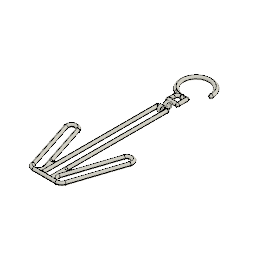
shoe-hanger v3 (Autodesk Fusion 360 design; units mm, degrees)
Autodesk Fusion 360 part; units mm, degrees
sketch "Sketch1" plane through (0, 0, 0) normal (0, 0, 1) x (1, 0, 0) in component "shoe holder"
  line L0 (67.4979, 112.1793) -> (43.75, 119.9918)
  line L1 (43.75, 119.9918) -> (12.5, 25)
  line L2 (12.5, 225) -> (-12.5, 225)
  line L3 (-12.5, 225) -> (-12.5, 25)
  line L4 (12.5, 25) -> (12.5, 225)
  line L5 (30.5937, 0) -> (-30.5937, 0)
  line L6 (0, 225) -> (0, 0) construction
  line L7 (67.4979, 112.1793) -> (30.5937, 0)
  line L8 (-67.4979, 112.1793) -> (-43.75, 119.9918)
  line L9 (-43.75, 119.9918) -> (-12.5, 25)
  line L10 (-67.4979, 112.1793) -> (-30.5937, 0)
  dimension "d8" = 25
  dimension "d11" = 25
  dimension "d14" = 200
  dimension "d56" = 100
  dimension "d57" = 100
  dimension "d58" = 31.25
  dimension "d59" = 25
  constraint horizontal L2
  constraint perpendicular L2 L3
  constraint parallel L3 L4
  constraint horizontal L5
  constraint midpoint L2 L6.start
  constraint coincident L6.end origin
  constraint symmetric L0.start L6 L8.start
  constraint symmetric L0.end L6 L8.end
  constraint parallel L9 L10
  constraint parallel L1 L7
  constraint perpendicular L0 L1
  constraint perpendicular L8 L9
  constraint coincident L1.end L4.start
  constraint midpoint L5 L6.end
  constraint coincident L3.end L9.end
  measures "d8" distance of L3.end L1.end
  measures "d11" distance of L0.start L0.end
  measures "d14" distance of L2.start L1.end
  measures "d56" distance of L0.end L1.end
  measures "d57" distance of L3.end L8.end
  measures "d58" distance of L0.end L4
  measures "d59" distance of L1.end L5
extrude "Extrude1" add sketch "Sketch1" along normal blind 8 makes body 1 in component "shoe holder"
fillet "Fillet1" radius 12.5 6 edges at (-67.4979, 112.1793, 4) (-43.75, 119.9918, 4) (-30.5937, 0, 4) (30.5937, 0, 4) (67.4979, 112.1793, 4) (43.75, 119.9918, 4) on bodies 1 in component "shoe holder"
fillet "Fillet1" radius 1.3333 2 edges at (-12.5, 25, 4) (12.5, 25, 4) on bodies 1 in component "shoe holder"
sketch "Sketch3" plane through (0, 0, 8) normal (0, 0, 1) x (-1, 0, 0) in component "shoe holder"
  arc A0 (-21.5468, 0) -> (-33.4208, -8.5938) centre (-21.5468, -12.5) ccw
  line L0 (-33.4208, -8.5938) -> (-63.5917, -100.3053)
  line L1 (-39.8438, -108.1178) -> (-15.0999, -32.903)
  line L2 (-12.5, -33.3196) -> (-12.5, -225)
  line L3 (12.5, -225) -> (12.5, -33.3196)
  line L4 (15.0999, -32.903) -> (39.8437, -108.1178)
  arc A1 (39.8437, -108.1178) -> (63.5917, -100.3053) centre (51.7177, -104.2116) ccw
  line L5 (63.5917, -100.3053) -> (33.4208, -8.5938)
  arc A2 (33.4208, -8.5938) -> (21.5468, 0) centre (21.5468, -12.5) ccw
  line L6 (21.5468, 0) -> (-21.5468, 0)
  arc A3 (26.2964, -10.9375) -> (16.7972, -14.0625) centre (21.5468, -12.5) ccw
  arc A4 (-21.5468, -7.5) -> (-26.2964, -10.9375) centre (-21.5468, -12.5) ccw
  line L7 (-26.2964, -10.9375) -> (-56.4673, -102.6491)
  arc A5 (-56.4673, -102.6491) -> (-46.9681, -105.7741) centre (-51.7177, -104.2116) ccw
  arc A6 (46.9681, -105.7741) -> (56.4673, -102.6491) centre (51.7177, -104.2116) ccw
  line L8 (56.4673, -102.6491) -> (26.2964, -10.9375)
  line L9 (46.9681, -105.7741) -> (16.7972, -14.0625)
  line L10 (-46.9681, -105.7741) -> (-16.7972, -14.0625)
  arc A7 (-16.7972, -14.0625) -> (-26.2964, -10.9375) centre (-21.5468, -12.5) ccw
  arc A8 (26.2964, -10.9375) -> (16.7972, -14.0625) centre (21.5468, -12.5) ccw
  arc A9 (-63.5917, -100.3053) -> (-39.8438, -108.1178) centre (-51.7177, -104.2116) ccw
  arc A10 (-12.5, -33.3196) -> (-15.0999, -32.903) centre (-13.8333, -33.3196) ccw
  arc A11 (15.0999, -32.903) -> (12.5, -33.3196) centre (13.8333, -33.3196) ccw
  dimension "d37" = 10
  dimension "d38" = 10
  constraint tangent A6 L9
  constraint tangent A5 L10
  constraint concentric A2 A3
  constraint concentric A0 A4
  constraint parallel L0 L7
  constraint concentric A1 A6
  constraint parallel L5 L8
  constraint tangent A3 L8
  constraint tangent A4 L7
  constraint tangent L7 A5
  constraint tangent A6 L8
  constraint concentric A3 A8
  constraint tangent L9 A8
  constraint concentric A4 A7
  measures "d37" distance of L8 L9
  measures "d38" distance of L7 L10
extrude "Extrude3" cut sketch "Sketch3" against normal through all bodies 1 in component "shoe holder"
sketch "Sketch4" plane through (0, 0, 8) normal (0, 0, 1) x (-1, 0, 0) in component "shoe holder"
  line L0 (46.9681, -105.7741) -> (16.7972, -14.0625)
  arc A0 (26.2964, -10.9375) -> (16.7972, -14.0625) centre (21.5468, -12.5) ccw
  line L1 (26.2964, -10.9375) -> (56.4673, -102.6491)
  arc A1 (46.9681, -105.7741) -> (56.4673, -102.6491) centre (51.7177, -104.2116) ccw
  line L2 (-16.7972, -14.0625) -> (-46.9681, -105.7741)
  arc A2 (-56.4673, -102.6491) -> (-46.9681, -105.7741) centre (-51.7177, -104.2116) ccw
  line L3 (-56.4673, -102.6491) -> (-26.2964, -10.9375)
  arc A3 (-16.7972, -14.0625) -> (-26.2964, -10.9375) centre (-21.5468, -12.5) ccw
  arc A4 (-21.5468, 0) -> (-33.4208, -8.5938) centre (-21.5468, -12.5) ccw
  line L4 (-33.4208, -8.5938) -> (-63.5917, -100.3053)
  line L5 (-39.8438, -108.1178) -> (-15.0999, -32.903)
  line L6 (-12.5, -33.3196) -> (-12.5, -225)
  line L7 (-12.5, -225) -> (12.5, -225)
  line L8 (12.5, -225) -> (12.5, -33.3196)
  line L9 (15.0999, -32.903) -> (39.8437, -108.1178)
  arc A5 (39.8437, -108.1178) -> (63.5917, -100.3053) centre (51.7177, -104.2116) ccw
  line L10 (63.5917, -100.3053) -> (33.4208, -8.5938)
  arc A6 (33.4208, -8.5938) -> (21.5468, 0) centre (21.5468, -12.5) ccw
  line L11 (21.5468, 0) -> (-21.5468, 0)
  line L12 (-4.5, -217) -> (4.5, -217)
  line L13 (-4.5, -217) -> (-4.5, -8)
  line L14 (4.5, -8) -> (-4.5, -8)
  line L15 (4.5, -217) -> (4.5, -8)
  arc A7 (-63.5917, -100.3053) -> (-39.8438, -108.1178) centre (-51.7177, -104.2116) ccw
  arc A8 (-12.5, -33.3196) -> (-15.0999, -32.903) centre (-13.8333, -33.3196) ccw
  arc A9 (15.0999, -32.903) -> (12.5, -33.3196) centre (13.8333, -33.3196) ccw
  dimension "d42" = 8
  dimension "d43" = 8
  dimension "d44" = 8
  dimension "d45" = 8
  constraint parallel L7 L12
  constraint perpendicular L13 L14
  constraint perpendicular L14 L15
  measures "d42" distance of L7 L12
  measures "d43" distance of L6 L13
  measures "d44" distance of L8 L15
  measures "d45" distance of L11 L14
extrude "Extrude4" cut sketch "Sketch4" against normal through all contours L12 L13 L14 L15 bodies 1 in component "shoe holder"
fillet "Fillet4" radius 4 4 edges at (0, 217, 8) (0, 217, 0) (0, 8, 8) (0, 8, 0) on bodies 1 in component "shoe holder"
fillet "Fillet4" radius 3.7383 4 edges at (-4.5, 112.5, 8) (4.5, 112.5, 8) (-4.5, 112.5, 0) (4.5, 112.5, 0) 18 faces at (12.5, 97.212, 2.6667) (12.808, 32.4658, 2.6667) (31.5961, 83.0473, 2.6667) (56.1868, 115.8855, 2.6667) (55.6248, 116.0853, 2.6667) (42.1464, 112.2526, 2.6667) (53.5351, 69.7358, 5.3333) (22.1284, 0.0135, 2.6667) (7.1829, 0, 2.6667) (-30.4167, 3.6915, 2.6667) (-53.5351, 69.7358, 5.3333) (-57.8025, 115.1311, 2.6667) (-55.6248, 116.0853, 2.6667) (-42.1464, 112.2526, 2.6667) (-31.5961, 83.0473, 2.6667) (-14.9586, 32.6037, 2.6667) (-12.5, 161.106, 2.6667) (4.1667, 225, 2.6667) on bodies 1 in component "shoe holder"
fillet "Fillet4" radius 3.7383 8 faces at (-46.4103, 72.0785, 5.3333) (-55.0954, 107.8982, 2.6667) (-36.9112, 75.2035, 5.3333) (-22.0761, 7.5281, 2.6667) (36.9112, 75.2035, 5.3333) (56.7013, 104.6167, 2.6667) (36.3534, 41.508, 5.3333) (18.1692, 8.8134, 5.3333) on bodies 1 in component "shoe holder"
sketch "Sketch5" plane through (0, 0, 0) normal (1, 0, 0) x (0, 1, 0) in component "hook"
  line L0 (221, 4) -> (223.1376, 9.8731) construction
  line L1 (221, 4) -> (231.5, 4) construction
  arc A0 (223.1376, 9.8731) -> (227.25, 4) centre (221, 4) ccw
  arc A1 (222.4536, 7.9937) -> (225.25, 4) centre (221, 4) ccw
  arc A2 (230.0464, 0.0063) -> (227.25, 4) centre (231.5, 4) ccw
  line L2 (223.1376, 9.8731) -> (222.4536, 7.9937)
  arc A3 (229.3624, -1.8731) -> (225.25, 4) centre (231.5, 4) ccw
  line L3 (230.0464, 0.0063) -> (229.3624, -1.8731)
  line L4 (231.5, 4) -> (229.3624, -1.8731) construction
  point P0 (225.25, 4)
  dimension "d103" = 8.5
  dimension "d104" = 221
  dimension "d105" = 4
  dimension "d111" = 70
  dimension "d113" = 2
  dimension "d114" = 2
  dimension "d116" = 4.25
  dimension "d117" = 70
  constraint coincident L0.start L1.start
  constraint coincident L1.end A2.centre
  constraint horizontal L1
  constraint coincident L1 P0
  constraint coincident P0 A1
  constraint coincident P0 A1.end
  constraint concentric A0 A1
  constraint coincident L0 A1.start
  constraint coincident L1 A0.end
  constraint parallel L3 L4
  measures "d103" diameter of A1
  measures "d104" horizontal distance of origin L0.start
  measures "d105" vertical distance of origin L0.start
  measures "d111" angle of L0 L1
  measures "d113" distance of A0 A1
  measures "d116" radius of A2
  measures "d117" angle of L1 L4
extrude "Extrude1'" add sketch "Sketch5" along normal mid plane 8 separate body makes body 2 in component "hook"
sketch "Sketch1 (2)" plane through (0, 0, 0) normal (0, 0, 1) x (1, 0, 0) in component "hanger"
  line L0 (0, 263) -> (12.5, 263)
  line L1 (12.5, 263) -> (12.5, 238)
  line L2 (12.5, 238) -> (-12.5, 238)
  line L3 (-12.5, 238) -> (-12.5, 257.6791)
  line L4 (0, 0) -> (0, 238)
  line L5 (4.5, 246) -> (-4.5, 246)
  line L6 (-4.5, 246) -> (-4.5, 255)
  line L7 (-4.5, 255) -> (4.5, 255)
  line L8 (4.5, 255) -> (4.5, 246)
  line L9 (0, 285.5) -> (30.3839, 282.8417) construction
  arc A0 (30.3839, 282.8417) -> (-12.5, 257.6791) centre (0, 285.5) ccw
  arc A1 (22.4144, 283.539) -> (0, 263) centre (0, 285.5) ccw
  line L10 (22.4144, 283.539) -> (30.3839, 282.8417)
  point P0 (0, 255)
  dimension "d86" = 238
  dimension "d89" = 45
  dimension "d91" = 85
  dimension "d92" = 25
  dimension "d93" = 25
  dimension "d94" = 8
  dimension "d95" = 8
  dimension "d96" = 8
  dimension "d97" = 8
  dimension "d98" = 8
  constraint horizontal L0
  constraint vertical L1
  constraint horizontal L2
  constraint vertical L3
  constraint coincident L4.start origin
  constraint midpoint L2 L4.end
  constraint vertical L4
  constraint vertical L9.start L0.start
  constraint coincident L9.start A0.centre
  constraint concentric A0 A1
  constraint coincident L9 A1.start
  constraint parallel L2 L5
  constraint parallel L3 L6
  constraint parallel L0 L7
  constraint parallel L1 L8
  constraint midpoint L7 P0
  constraint vertical L0.start P0
  measures "d86" distance of L4.start L4.end
  measures "d89" diameter of A1
  measures "d91" angle of L0.start L9.start L9.end
  measures "d92" distance of L0.end L1.end
  measures "d93" distance of L1.end L2.end
  measures "d94" distance of A0 A1
  measures "d95" distance of L1 L8
  measures "d96" distance of L2 L5
  measures "d97" distance of L3 L6
  measures "d98" distance of L0 L7
extrude "Extrude1''" add sketch "Sketch1 (2)" along normal blind 8 separate body makes body 3 in component "hanger"
fillet "Fillet1'" radius 3.9801 24 edges at (6.25, 263, 8) (-15.2008, 302.0887, 8) (-15.4353, 311.8059, 8) (-15.4353, 311.8059, 0) (-15.2008, 302.0887, 0) (6.25, 263, 0) (-12.5, 247.8396, 0) (-12.5, 247.8396, 8) (-12.5, 238, 4) (0, 238, 0) (12.5, 238, 4) (12.5, 250.5, 0) (12.5, 250.5, 8) (12.5, 263, 4) (-12.5, 257.6791, 4) (0, 255, 8) (0, 255, 0) (0, 246, 8) (0, 246, 0) (-4.5, 250.5, 8) (-4.5, 250.5, 0) (4.5, 250.5, 8) (4.5, 250.5, 0) (0, 238, 8) 1 faces at (25.0709, 283.3066, 2.6667) on bodies 3 in component "hanger"
fillet "Fillet1'" radius 4 2 edges at (-4.5, 255, 4) (4.5, 255, 4) on bodies 3 in component "hanger"
fillet "Fillet2" radius 1 2 faces at (4, 230.6971, -1.5107) (-4, 230.6971, -1.5107) on bodies 2 in component "hook"
fillet "Fillet2" radius 1 2 faces at (1.3333, 229.5904, -1.2466) (1.3333, 222.6816, 8.6202) on bodies 2 in component "hook"
component "shoe holder" placed x (1, 0, 0) y (0, 1, 0) z (0, 0, 1) at (0, 0, 0)
component "hook" placed x (1, 0, 0) y (0, 1, 0) z (0, 0, 1) at (0, 0, 0)
component "hanger" placed x (1, 0, 0) y (0, 1, 0) z (0, 0, 1) at (0, 0, 0)
equation "mid_to_shoe = 60 mm"
equation "heel_to_toe = 100 mm"
equation "heel_to_hook = 200 mm"
equation "d8 = width"
equation "d11 = width"
equation "d14 = heel_to_hook"
equation "width = 25 mm"
equation "thick = 8 mm"
equation "d22 = thick"
equation "d25 = width / 2"
equation "d42 = thick"
equation "d43 = thick"
equation "d44 = thick"
equation "d45 = thick"
equation "d56 = heel_to_toe"
equation "d57 = heel_to_toe"
equation "d58 = width * 1.25"
equation "d59 = width"
equation "d61 = thick / 6"
equation "d63 = thick / 2"
equation "d65 = thick / 2.14"
equation "d67 = thick / 2.14"
equation "hanger_diam = 45 mm"
equation "d89 = hanger_diam"
equation "d92 = width"
equation "d93 = width"
equation "d94 = thick"
equation "d95 = thick"
equation "d96 = thick"
equation "d97 = thick"
equation "d98 = thick"
equation "d99 = thick"
equation "d102 = thick / 2.01"
equation "d103 = thick + 0.5 mm"
equation "d116 = d103 / 2"
equation "d117 = d111"
equation "d118 = thick"
equation "d121 = thick / 2"
named bodies: "holder", "hanger", "hook"
